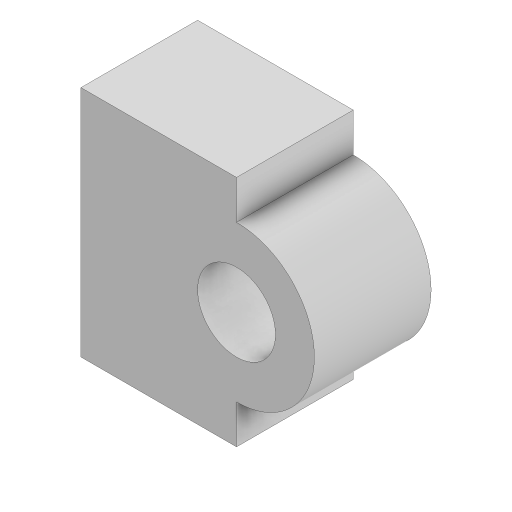
# Autodesk Inventor part: RODAMIENTO DE TORNILLO
Saved by Autodesk Inventor 2024 (Build 280153000, 153)
## iProperties
Created: 2024-06-13
Part Number: RODAMIENTO DE TORNILLO
Material: Generic
Document SubType Name: Modeling
Designer: Jhuliams
Density: 1 g/cm^3
Appearance: Default
Author: Jhuliams
Autodesk Inventor part; units mm, degrees
ref_plane "YZ Plane" through (0, 0, 0) normal (1, 0, 0) x (0, 1, 0)
ref_plane "XZ Plane" through (0, 0, 0) normal (0, 1, 0) x (-1, 0, 0)
ref_plane "XY Plane" through (0, 0, 0) normal (0, 0, 1) x (1, 0, 0)
sketch "Sketch1" plane through (0, 0, 0) normal (0, 0, 1) x (1, 0, 0)
  circle A0 centre (0, 0) radius 5
  line L0 (0, 0) -> (-20, 0) construction
  line L1 (-20, 0) -> (-20, -15)
  line L2 (-20, -15) -> (0, -15)
  line L3 (0, -15) -> (0, -5)
  circle A1 centre (0, 0) radius 10
  line L4 (-20, 0) -> (-20, 15)
  line L5 (-20, 15) -> (0, 15)
  line L6 (0, 15) -> (0, 5)
  point P0 (0, -10)
  point P1 (0, 10)
  dimension "d0" = 10
  dimension "d1" = 20
  dimension "d2" = 15
  dimension "d3" = 20
  constraints: 14 end point, 3 symmetric about line, 2 coincident, 2 perpendicular, 1 centre point, 1 horizontal, 1 vertical, 1 vertical alignment, 2 other
  measures "d1" distance of L0.start L0.end
  measures "d2" distance of L0.end L1.end
  measures "d3" diameter of A1
extrude "Extrusion1" add sketch "Sketch1" along normal mid plane 15 contours A0 L6 A1 L3 | A0 L3 A1 L6 | A1 L3 L2 L1 L4 L5 L6
body "Solid1"
